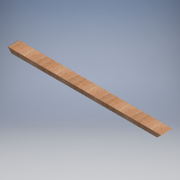
# Autodesk Inventor part: Right Panel Rear 45 Diagonal Piece
Saved by Autodesk Inventor 2016 (Build 200138000, 138)
## iProperties
Created: 2015-07-05
Part Number: Right Panel Rear 45 Diagonal Piece
Material: Wood (Birch)
Document SubType Name: Modeling
Designer: steele
Density: 0.55 g/cm^3
Appearance: Birch - Natural Polished
Author: steele
Autodesk Inventor part; units mm, degrees
ref_plane "YZ Plane" through (0, 0, 0) normal (1, 0, 0) x (0, 1, 0)
ref_plane "XZ Plane" through (0, 0, 0) normal (0, 1, 0) x (-1, 0, 0)
ref_plane "XY Plane" through (0, 0, 0) normal (0, 0, 1) x (1, 0, 0)
sketch "Sketch2" plane through (0, 0, 0) normal (0, 0, 1) x (1, 0, 0)
  line L0 (-577.2629, -20.1175) -> (572.0871, -20.1175)
  line L1 (610.1871, 17.9825) -> (-615.3629, 17.9825)
  line L2 (-615.2407, -18.1315) -> (610.1871, 17.9825) construction
  line L3 (610.0737, -17.828) -> (-615.3629, 17.9825) construction
  line L4 (-615.3629, 17.9825) -> (-577.2629, -20.1175)
  line L5 (-615.3629, 17.9825) -> (-561.4814, 17.9825) construction
  line L6 (610.1871, 17.9825) -> (572.0871, -20.1175)
  line L7 (610.1871, 17.9825) -> (664.0686, 17.9825) construction
  point P0 (0, 0)
  dimension "d10" = 45
  dimension "d11" = 135
  dimension "d14" = 1225.55
  dimension "d15" = 38.1
  constraints: 16 end point, 3 horizontal, 2 equal length, 2 point on line, 1 parallel
  measures "d10" angle of L4 L5
  measures "d11" angle of L6 L7
  measures "d14" distance of L1.start L1.end
  measures "d15" distance between parallel lines of L0 L1
extrude "Extrusion2" add sketch "Sketch2" along normal mid plane 88.9
body "Solid2"
